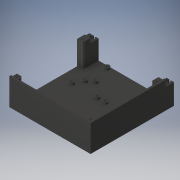
# Autodesk Inventor part: Base Right No Front Panel Or Back Panel
Saved by Autodesk Inventor 2019 (Build 230136000, 136)
## iProperties
Created: 2018-11-05
Part Number: Base Right No Front Panel Or Back Panel
Material: Generic
Document SubType Name: Modeling
Designer: Keith
Density: 1 g/cm^3
Appearance: Default
Author: Keith
## iProperties of the stored document Base Right No Front Panel_3DPrint.ipt
Created: 2018-12-04
Part Number: Base Right No Front Panel_3DPrint
Material: Generic
Document SubType Name: Modeling
Designer: Keith
Density: 1 g/cm^3
Appearance: Default
Author: Keith
Autodesk Inventor part; units mm, degrees
ref_plane "YZ Plane" through (0, 0, 0) normal (1, 0, 0) x (0, 1, 0)
ref_plane "XZ Plane" through (0, 0, 0) normal (0, 1, 0) x (-1, 0, 0)
sketch "Sketch1" plane through (0, 0, 0) normal (0, 1, 0) x (-1, 0, 0)
  line L0 (0, 0) -> (124, 0)
  line L1 (124, 0) -> (124, -124.8)
  line L2 (0, -124.8) -> (0, 0)
  line L3 (113, -2.5) -> (11, -2.5)
  line L4 (124, 0) -> (113, 0)
  line L5 (113, -2.5) -> (113, -11.25)
  line L6 (113, -11.25) -> (121.5, -11.25)
  line L7 (124, -11.25) -> (124, 0)
  line L8 (0, 0) -> (11, 0)
  line L9 (11, -2.5) -> (11, -11.25)
  line L10 (11, -11.25) -> (2.5, -11.25)
  line L11 (0, -11.25) -> (0, 0)
  line L12 (113, -112.8) -> (121.5, -112.8)
  line L13 (124, -112.8) -> (124, -124.8)
  line L14 (11, -112.8) -> (2.5, -112.8)
  line L15 (0, -112.8) -> (0, -124.8)
  line L16 (2.5, -112.8) -> (11, -112.8)
  line L17 (11, -112.8) -> (11, -101.55)
  line L18 (11, -101.55) -> (2.5, -101.55)
  line L19 (0, -101.55) -> (0, -112.8)
  line L20 (113, -112.8) -> (121.5, -112.8)
  line L21 (124, -112.8) -> (124, -101.55)
  line L22 (121.5, -101.55) -> (113, -101.55)
  line L23 (113, -101.55) -> (113, -112.8)
  line L24 (2.5, -11.25) -> (2.5, -101.55)
  line L25 (2.5, -112.8) -> (2.5, -122.3)
  line L26 (121.5, -122.3) -> (121.5, -112.8)
  line L27 (121.5, -101.55) -> (121.5, -11.25)
  line L28 (121.5, -122.3) -> (121.5, -124.8)
  line L29 (2.5, -122.3) -> (2.5, -124.8)
  line L30 (124, -124.8) -> (121.5, -124.8)
  line L31 (2.5, -124.8) -> (0, -124.8)
  dimension "d1" = 124.8
  dimension "d3" = 2.5
  dimension "d6" = 11
  dimension "d7" = 11.25
  dimension "d8" = 11
  dimension "d9" = 11.25
  dimension "d10" = 11
  dimension "d12" = 11
  dimension "d14" = 11
  dimension "d15" = 11.25
  dimension "d16" = 11.25
  constraints: 64 end point, 15 parallel, 9 perpendicular, 6 horizontal, 1 point on line
  measures "d1" distance of L0.end L1.end
  measures "d3" distance between parallel lines of L0 L3
  measures "d6" distance of L7.start L5.end
  measures "d7" distance of L5.end L4.end
  measures "d8" distance of L9.end L11.start
  measures "d9" distance of L8.end L9.end
  measures "d10" distance of L12.start L13.start
  measures "d12" distance of L15.start L14.start
  measures "d14" distance of L19.start L17.end
  measures "d15" distance of L17.end L16.end
  measures "d16" distance of L21.end L21.start
extrude "Extrusion1" add sketch "Sketch1" along normal blind 43
sketch "Sketch2" plane through (0, 0, 0) normal (0, -1, 0) x (1, 0, 0)
  line L0 (0, 0) -> (0, -124.8) projected
  line L1 (-124, 0) -> (0, 0) projected
  line L2 (-124, -124.8) -> (-124, 0) projected
  line L3 (-121.5, -124.8) -> (-124, -124.8) projected
  line L4 (-121.5, -112.8) -> (-121.5, -124.8) projected
  line L5 (-113, -112.8) -> (-121.5, -112.8) projected
  line L6 (-113, -101.55) -> (-113, -112.8) projected
  line L7 (-121.5, -101.55) -> (-113, -101.55) projected
  line L8 (-121.5, -11.25) -> (-121.5, -101.55) projected
  line L9 (-113, -11.25) -> (-121.5, -11.25) projected
  line L10 (-113, -2.5) -> (-113, -11.25) projected
  line L11 (-11, -2.5) -> (-113, -2.5) projected
  line L12 (-11, -11.25) -> (-11, -2.5) projected
  line L13 (-2.5, -11.25) -> (-11, -11.25) projected
  line L14 (-2.5, -101.55) -> (-2.5, -11.25) projected
  line L15 (-11, -101.55) -> (-2.5, -101.55) projected
  line L16 (-11, -112.8) -> (-11, -101.55) projected
  line L17 (-2.5, -112.8) -> (-11, -112.8) projected
  line L18 (-2.5, -124.8) -> (-2.5, -112.8) projected
  line L19 (0, -124.8) -> (-2.5, -124.8) projected
  line L20 (-124, -124.8) -> (0, -124.8)
  line L21 (0, -124.8) -> (0, 0)
  line L22 (0, 0) -> (-124, 0)
  line L23 (-124, 0) -> (-124, -124.8)
  constraints: 8 end point, 2 parallel, 1 horizontal, 1 perpendicular
extrude "Extrusion2" add sketch "Sketch2" against normal blind 2
sketch "Sketch3" plane through (0, 2, 0) normal (0, 1, 0) x (1, 0, 0)
  line L0 (-121.5, 112.8) -> (-121.5, 124.8) projected
  line L1 (-113, 112.8) -> (-121.5, 112.8) projected
  line L2 (-113, 101.55) -> (-113, 112.8) projected
  line L3 (-121.5, 101.55) -> (-113, 101.55) projected
  line L4 (-121.5, 11.25) -> (-121.5, 101.55) projected
  line L5 (-113, 11.25) -> (-121.5, 11.25) projected
  line L6 (-113, 2.5) -> (-113, 11.25) projected
  line L7 (-11, 2.5) -> (-113, 2.5) projected
  line L8 (-11, 11.25) -> (-11, 2.5) projected
  line L9 (-2.5, 11.25) -> (-11, 11.25) projected
  line L10 (-2.5, 101.55) -> (-2.5, 11.25) projected
  line L11 (-11, 101.55) -> (-2.5, 101.55) projected
  line L12 (-11, 112.8) -> (-11, 101.55) projected
  line L13 (-2.5, 112.8) -> (-11, 112.8) projected
  line L14 (-2.5, 124.8) -> (-2.5, 112.8) projected
  line L15 (-2.5, 124.8) -> (-121.5, 124.8) projected
  line L16 (-11, 112.8) -> (-2.5, 112.8)
  line L17 (-2.5, 112.8) -> (-2.5, 124.8)
  line L18 (-2.5, 124.8) -> (-11, 124.8)
  line L19 (-11, 124.8) -> (-11, 112.8)
  line L20 (-113, 112.8) -> (-121.5, 112.8)
  line L21 (-121.5, 112.8) -> (-121.5, 124.8)
  line L22 (-121.5, 124.8) -> (-113, 124.8)
  line L23 (-113, 124.8) -> (-113, 112.8)
  point P0 (0, 0)
  constraints: 16 end point, 4 parallel, 2 horizontal, 2 perpendicular
extrude "Extrusion3" add sketch "Sketch3" along normal blind 30.6 contours L0 L15 L23 L1 | L15 L14 L13 L19
sketch "Sketch4" plane through (0, 0, -124.8) normal (1, 0, 0) x (0, 0, -1)
  line L0 (0, 32.6) -> (-12, 32.6) projected
  line L1 (-12, 32.6) -> (-12, 43) projected
  line L2 (-124.8, 43) -> (0, 43) projected
  line L3 (0, 0) -> (0, 43) projected
  point P0 (-124.8, 0)
extrude "Extrusion4" cut sketch "Sketch4" against normal through all
sketch "Sketch5" plane through (0, 43, 0) normal (0, 1, 0) x (1, 0, 0)
  line L0 (-113, 112.8) -> (-124, 112.8) projected
  line L1 (-124, 112.8) -> (-124, 0) projected
  line L2 (-124, 0) -> (0, 0) projected
  line L3 (0, 0) -> (0, 112.8) projected
  line L4 (0, 112.8) -> (-11, 112.8) projected
  line L5 (-11, 112.8) -> (-11, 101.55) projected
  line L6 (-11, 101.55) -> (-2.5, 101.55) projected
  line L7 (-2.5, 101.55) -> (-2.5, 11.25) projected
  line L8 (-2.5, 11.25) -> (-11, 11.25) projected
  line L9 (-11, 11.25) -> (-11, 2.5) projected
  line L10 (-11, 2.5) -> (-113, 2.5) projected
  line L11 (-113, 2.5) -> (-113, 11.25) projected
  line L12 (-113, 11.25) -> (-121.5, 11.25) projected
  line L13 (-121.5, 11.25) -> (-121.5, 101.55) projected
  line L14 (-121.5, 101.55) -> (-113, 101.55) projected
  line L15 (-113, 101.55) -> (-113, 112.8) projected
  circle A0 centre (-6.625, 6.875) radius 1.35
  circle A1 centre (-6.625, 105.8) radius 1.35
  line L16 (-62, 2.5) -> (-62, 12.6966)
  line L17 (0, 0) -> (-124, 0)
  line L18 (-124, 0) -> (-124, 112.8)
  line L19 (-124, 112.8) -> (-113, 112.8)
  line L20 (-113, 112.8) -> (-113, 101.55)
  line L21 (-113, 101.55) -> (-121.5, 101.55)
  line L22 (-121.5, 101.55) -> (-121.5, 11.25)
  line L23 (-121.5, 11.25) -> (-113, 11.25)
  line L24 (-113, 11.25) -> (-113, 2.5)
  line L25 (-113, 2.5) -> (-11, 2.5)
  circle A2 centre (-117.375, 6.875) radius 1.35
  circle A3 centre (-117.375, 105.8) radius 1.35
  dimension "d25" = 2.7
  dimension "d26" = 4.375
  dimension "d27" = 4.375
  dimension "d28" = 2.7
  dimension "d29" = 4.25
  dimension "d30" = 4.375
  constraints: 20 end point, 7 symmetric about line, 4 centre point, 1 midpoint, 1 vertical, 2 other
  measures "d25" diameter of A0
  measures "d26" distance from line of L8 A0.centre
  measures "d27" distance from line of L9 A0.centre
  measures "d28" diameter of A1
  measures "d29" distance from line of L6 A1.centre
  measures "d30" distance from line of L5 A1.centre
extrude "Extrusion5" cut sketch "Sketch5" against normal blind 12 contours A0 | A1 | A2 | A3
sketch "Sketch6" plane through (0, 0, 0) normal (1, 0, 0) x (0, 0, -1)
  line L0 (0, 43) -> (112.8, 43) projected
  line L1 (0, 0) -> (0, 43) projected
  line L2 (0, 0) -> (124.8, 0) projected
  line L3 (124.8, 0) -> (124.8, 32.6) projected
  line L4 (112.8, 32.6) -> (112.8, 43) projected
  line L5 (124.8, 0) -> (124.8, 32.6) projected
  line L6 (112.8, 32.6) -> (124.8, 32.6)
  line L7 (124.8, 32.6) -> (124.8, 30.6)
  line L8 (124.8, 30.6) -> (112.8, 30.6)
  line L9 (112.8, 30.6) -> (112.8, 32.6)
  line L10 (124.8, 32.6) -> (112.8, 32.6) projected
  line L11 (112.8, 32.6) -> (112.8, 43) projected
  dimension "d33" = 30.6
  constraints: 8 end point, 2 parallel, 1 horizontal, 1 perpendicular, 1 point on line
  measures "d33" distance between parallel lines of L2 L8
extrude "Extrusion6" cut sketch "Sketch6" against normal through all contours L6 L3 L8 L9
sketch "Sketch7" plane through (0, 43, 0) normal (0, 1, 0) x (1, 0, 0)
  circle A0 centre (-6.625, 6.875) radius 1.35 projected
  circle A1 centre (-117.375, 105.8) radius 1.35 projected
  circle A2 centre (-6.625, 6.875) radius 1.35 projected
  circle A3 centre (-6.625, 105.8) radius 1.35 projected
  circle A4 centre (-117.375, 6.875) radius 1.35 projected
  line L0 (-113, 112.8) -> (-124, 112.8) projected
  line L1 (-124, 112.8) -> (-124, 0) projected
  line L2 (-124, 0) -> (0, 0) projected
  line L3 (0, 0) -> (0, 112.8) projected
  line L4 (0, 112.8) -> (-11, 112.8) projected
  line L5 (-11, 112.8) -> (-11, 101.55) projected
  line L6 (-11, 101.55) -> (-2.5, 101.55) projected
  line L7 (-2.5, 101.55) -> (-2.5, 11.25) projected
  line L8 (-2.5, 11.25) -> (-11, 11.25) projected
  line L9 (-11, 11.25) -> (-11, 2.5) projected
  line L10 (-11, 2.5) -> (-113, 2.5) projected
  line L11 (-113, 2.5) -> (-113, 11.25) projected
  line L12 (-113, 11.25) -> (-121.5, 11.25) projected
  line L13 (-121.5, 11.25) -> (-121.5, 101.55) projected
  line L14 (-121.5, 101.55) -> (-113, 101.55) projected
  line L15 (-113, 101.55) -> (-113, 112.8) projected
extrude "Extrusion7" cut sketch "Sketch7" against normal blind 3
sketch "Sketch8" plane through (0, 30.6, -112.8) normal (0, 1, 0) x (1, 0, 0)
  line L0 (-113, 12) -> (-113, 0) projected
  line L1 (-124, 12) -> (-113, 12) projected
  line L2 (-124, 0) -> (-124, 12) projected
  line L3 (-113, 0) -> (-124, 0) projected
  line L4 (-11, 0) -> (-11, 12) projected
  line L5 (0, 0) -> (-11, 0) projected
  line L6 (0, 12) -> (0, 0) projected
  line L7 (-11, 12) -> (0, 12) projected
  line L8 (-122.6, 10.6) -> (-122.6, 9.3834)
  line L9 (-120.075, 10.6) -> (-122.6, 10.6)
  line L10 (-122.6, 9.3834) -> (-120.0827, 6.9051)
  line L11 (-114.4, 10.6) -> (-114.4, 9.3834)
  line L12 (-116.925, 10.6) -> (-114.4, 10.6)
  line L13 (-114.4, 9.3834) -> (-116.9173, 6.9051)
  line L14 (-120, 12) -> (-117, 12)
  line L15 (-120.0827, 6.9051) -> (-116.9173, 6.9051)
  line L16 (-120.075, 10.6) -> (-120.075, 12)
  line L17 (-116.925, 10.6) -> (-116.925, 12)
  line L18 (-120.075, 12) -> (-120, 12)
  line L19 (0, 12) -> (-124, 12) projected
  line L20 (-117, 12) -> (-116.925, 12)
  point P0 (0, -112.8)
  point P1 (-114.4, 9.9917)
  constraints: 24 end point, 5 horizontal, 4 vertical, 3 collinear, 3 point on line, 1 midpoint, 3 other
extrude "Extrusion8" cut sketch "Sketch8" against normal through all contours L17 L12 L11 L13 L15 L10 L8 L9 L16 L1
ref_plane "Work Plane1" through (-62, 2, -101.55) normal (1, 0, 0) x (0, 0, -1)
mirror "Mirror1" about plane through (-62, 2, -101.55) normal (1, 0, 0) of "Extrusion8"
sketch "Sketch9" plane through (-124, 0, -124.8) normal (-1, 0, 0) x (0, 0, 1)
  line L0 (124.8, 40) -> (12, 40) projected
  line L1 (12, 40) -> (12, 30.6) projected
  line L2 (12, 30.6) -> (0, 30.6) projected
  line L3 (0, 0) -> (0, 30.6) projected
  line L4 (0, 0) -> (124.8, 0) projected
  line L5 (124.8, 0) -> (124.8, 40) projected
  line L6 (124.8, 40) -> (164.8, 40)
  line L7 (164.8, 40) -> (164.8, 0)
  line L8 (164.8, 0) -> (124.8, 0)
  line L9 (124.8, 0) -> (124.8, 40)
  circle A0 centre (134.8, 30) radius 2.6
  circle A1 centre (154.8, 30) radius 2.6
  circle A2 centre (154.8, 10) radius 2.6
  circle A3 centre (134.8, 10) radius 2.6
  dimension "d61" = 40
  dimension "d62" = 5.2
  dimension "d63" = 5.2
  dimension "d64" = 5.2
  dimension "d65" = 5.2
  dimension "d66" = 20
  dimension "d67" = 20
  dimension "d68" = 20
  dimension "d69" = 10
  dimension "d141" = 10
  dimension "d142" = 10
  dimension "d143" = 10
  constraints: 8 end point, 4 centre point, 2 parallel, 1 horizontal, 1 perpendicular
  measures "d61" distance of L7.end L8.end
  measures "d62" diameter of A0
  measures "d63" diameter of A1
  measures "d64" diameter of A2
  measures "d65" diameter of A3
  measures "d66" distance of A1.centre A0.centre
  measures "d67" distance of A2.centre A3.centre
  measures "d68" distance between centres of A1 A2
  measures "d69" distance from line of L8 A3.centre
  measures "d141" distance from line of L5 A0.centre
  measures "d142" distance from line of L6 A0.centre
  measures "d143" distance from line of L5 A3.centre
extrude "Extrusion9" add sketch "Sketch9" along normal blind 2.5
sketch "Sketch10" plane through (0, 2, 0) normal (0, 1, 0) x (1, 0, 0)
  line L0 (-113, 124.8) -> (-113, 101.55) projected
  line L1 (-121.5, 101.55) -> (-113, 101.55) projected
  line L2 (-121.5, 11.25) -> (-121.5, 101.55) projected
  line L3 (-113, 11.25) -> (-121.5, 11.25) projected
  line L4 (-113, 2.5) -> (-113, 11.25) projected
  line L5 (-11, 2.5) -> (-113, 2.5) projected
  line L6 (-11, 11.25) -> (-11, 2.5) projected
  line L7 (-2.5, 11.25) -> (-11, 11.25) projected
  line L8 (-2.5, 101.55) -> (-2.5, 11.25) projected
  line L9 (-11, 101.55) -> (-2.5, 101.55) projected
  line L10 (-11, 124.8) -> (-11, 101.55) projected
  line L11 (-11, 124.8) -> (-113, 124.8) projected
  circle A0 centre (-20.1, 87.8) radius 3.5
  circle A1 centre (-96.1, 87.8) radius 3.5
  line L12 (0, 112.8) -> (0, 0) projected
  circle A2 centre (-20.1, 87.8) radius 1.35
  circle A3 centre (-96.1, 87.8) radius 1.35
  dimension "d72" = 7
  dimension "d73" = 7
  dimension "d74" = 76
  dimension "d76" = 37
  dimension "d77" = 20.1
  dimension "d78" = 2.7
  dimension "d79" = 2.7
  constraints: 4 centre point, 2 coincident
  measures "d72" diameter of A0
  measures "d73" diameter of A1
  measures "d74" distance of A0.centre A1.centre
  measures "d76" distance from line of L11 A0.centre
  measures "d77" distance from line of L12 A0.centre
  measures "d78" diameter of A2
  measures "d79" diameter of A3
extrude "Extrusion10" add sketch "Sketch10" along normal blind 3 contours A0 | A1
sketch "Sketch11" plane through (0, 2, 0) normal (0, 1, 0) x (1, 0, 0)
  circle A0 centre (-20.1, 87.8) radius 1.35 projected
  circle A1 centre (-96.1, 87.8) radius 1.35 projected
  point P0 (0, 0)
extrude "Extrusion11" cut sketch "Sketch11" against normal blind 1
sketch "Sketch12" plane through (0, 2, 0) normal (0, 1, 0) x (1, 0, 0)
  circle A0 centre (-20.1, 87.8) radius 3.5 projected
  circle A1 centre (-96.1, 87.8) radius 3.5 projected
  line L0 (-113, 124.8) -> (-113, 101.55) projected
  line L1 (-121.5, 101.55) -> (-113, 101.55) projected
  line L2 (-121.5, 11.25) -> (-121.5, 101.55) projected
  line L3 (-113, 11.25) -> (-121.5, 11.25) projected
  line L4 (-113, 2.5) -> (-113, 11.25) projected
  line L5 (-11, 2.5) -> (-113, 2.5) projected
  line L6 (-11, 11.25) -> (-11, 2.5) projected
  line L7 (-2.5, 11.25) -> (-11, 11.25) projected
  line L8 (-2.5, 101.55) -> (-2.5, 11.25) projected
  line L9 (-11, 101.55) -> (-2.5, 101.55) projected
  line L10 (-11, 124.8) -> (-11, 101.55) projected
  line L11 (-11, 124.8) -> (-113, 124.8) projected
  circle A2 centre (-103, 12.5) radius 3.5
  circle A3 centre (-103, 75.3) radius 3.5
  circle A4 centre (-65.2, 12.5) radius 3.5
  circle A5 centre (-65.2, 75.3) radius 3.5
  circle A6 centre (-103, 12.5) radius 1.35
  circle A7 centre (-103, 75.3) radius 1.35
  circle A8 centre (-65.2, 75.3) radius 1.35
  circle A9 centre (-65.2, 12.5) radius 1.35
  line L12 (-59.1, 6.875) -> (-59.1, 19.1596)
  circle A10 centre (-15.2, 12.5) radius 3.5
  circle A11 centre (-15.2, 75.3) radius 3.5
  circle A12 centre (-53, 12.5) radius 3.5
  circle A13 centre (-53, 75.3) radius 3.5
  circle A14 centre (-15.2, 12.5) radius 1.35
  circle A15 centre (-15.2, 75.3) radius 1.35
  circle A16 centre (-53, 75.3) radius 1.35
  circle A17 centre (-53, 12.5) radius 1.35
  point P0 (0, 0)
  dimension "d84" = 7
  dimension "d85" = 7
  dimension "d86" = 7
  dimension "d87" = 7
  dimension "d88" = 62.8
  dimension "d89" = 62.8
  dimension "d90" = 37.8
  dimension "d91" = 10
  dimension "d92" = 10
  dimension "d93" = 2.7
  dimension "d94" = 2.7
  dimension "d95" = 2.7
  dimension "d96" = 2.7
  dimension "d97" = 6.1
  constraints: 16 centre point, 8 coincident, 8 symmetric about line, 2 end point, 1 vertical, 8 other
  measures "d84" diameter of A2
  measures "d85" diameter of A3
  measures "d86" diameter of A4
  measures "d87" diameter of A5
  measures "d88" distance of A3.centre A2.centre
  measures "d89" distance of A5.centre A4.centre
  measures "d90" distance of A4.centre A2.centre
  measures "d91" distance from line of L5 A2.centre
  measures "d92" distance from line of L4 A2.centre
  measures "d93" diameter of A6
  measures "d94" diameter of A7
  measures "d95" diameter of A8
  measures "d96" diameter of A9
  measures "d97" distance from line of A9.centre L12
extrude "Extrusion12" add sketch "Sketch12" along normal blind 3 contours A2 | A3 | A4 | A5 | A10 | A11 | A12 | A13
sketch "Sketch13" plane through (0, 2, 0) normal (0, 1, 0) x (1, 0, 0)
  circle A0 centre (-103, 12.5) radius 1.35 projected
  circle A1 centre (-103, 75.3) radius 1.35 projected
  circle A2 centre (-65.2, 75.3) radius 1.35 projected
  circle A3 centre (-65.2, 12.5) radius 1.35 projected
  circle A4 centre (-53, 12.5) radius 1.35 projected
  circle A5 centre (-53, 75.3) radius 1.35 projected
  circle A6 centre (-15.2, 75.3) radius 1.35 projected
  circle A7 centre (-15.2, 12.5) radius 1.35 projected
  point P0 (0, 0)
extrude "Extrusion13" cut sketch "Sketch13" against normal blind 1
sketch "Sketch15" plane through (0, 40, 0) normal (0, 1, 0) x (1, 0, 0)
  circle A0 centre (-117.375, 6.875) radius 1.35 projected
  circle A1 centre (-6.625, 105.8) radius 1.35 projected
  circle A2 centre (-117.375, 105.8) radius 1.35 projected
  circle A3 centre (-6.625, 6.875) radius 1.35 projected
  line L0 (-126.5, 112.8) -> (-113, 112.8) projected
  line L1 (-126.5, -40) -> (-126.5, 112.8) projected
  line L2 (-124, -40) -> (-126.5, -40) projected
  line L3 (-124, -40) -> (-124, 0) projected
  line L4 (0, 0) -> (-124, 0) projected
  line L5 (0, 112.8) -> (0, 0) projected
  line L6 (-11, 112.8) -> (0, 112.8) projected
  line L7 (-11, 101.55) -> (-11, 112.8) projected
  line L8 (-2.5, 101.55) -> (-11, 101.55) projected
  line L9 (-2.5, 11.25) -> (-2.5, 101.55) projected
  line L10 (-11, 11.25) -> (-2.5, 11.25) projected
  line L11 (-11, 2.5) -> (-11, 11.25) projected
  line L12 (-113, 2.5) -> (-11, 2.5) projected
  line L13 (-113, 11.25) -> (-113, 2.5) projected
  line L14 (-121.5, 11.25) -> (-113, 11.25) projected
  line L15 (-121.5, 101.55) -> (-121.5, 11.25) projected
  line L16 (-113, 101.55) -> (-121.5, 101.55) projected
  line L17 (-113, 112.8) -> (-113, 101.55) projected
  line L18 (-121.5, 2.5) -> (-2.5, 2.5)
  line L19 (-2.5, 2.5) -> (-2.5, 112.8)
  line L20 (-2.5, 112.8) -> (-121.5, 112.8)
  line L21 (-121.5, 112.8) -> (-121.5, 2.5)
  constraints: 8 end point, 2 parallel, 1 horizontal, 1 perpendicular, 1 point on line
extrude "Extrusion15" cut sketch "Sketch15" against normal blind 2.5 contours L0 L17 L16 L21 | L20 L7 L8 L9 L10 L11 L12 L13 L14 L15 L16 L17 | L6 L19 L8 L7 | L14 L13 L18 L21 | L19 L18 L11 L10
fillet "Fillet2" radius 3 4 edges at (-11, 19.75, -101.55) (-11, 19.75, -11.25) (-113, 19.75, -101.55) (-113, 19.75, -11.25)
sketch "Sketch16" plane through (0, 2, 0) normal (0, 1, 0) x (1, 0, 0)
  line L0 (-11, 124.8) -> (-113, 124.8) projected
  arc A0 (-8, 11.25) -> (-11, 8.25) centre (-8, 8.25) ccw projected
  line L1 (-2.5, 11.25) -> (-8, 11.25) projected
  line L2 (-2.5, 101.55) -> (-2.5, 11.25) projected
  line L3 (-8, 101.55) -> (-2.5, 101.55) projected
  arc A1 (-11, 104.55) -> (-8, 101.55) centre (-8, 104.55) ccw projected
  line L4 (-11, 124.8) -> (-11, 104.55) projected
  line L5 (-11, 124.8) -> (-113, 124.8) projected
  line L6 (-113, 124.8) -> (-113, 104.55) projected
  arc A2 (-116, 101.55) -> (-113, 104.55) centre (-116, 104.55) ccw projected
  line L7 (-121.5, 101.55) -> (-116, 101.55) projected
  line L8 (-121.5, 11.25) -> (-121.5, 101.55) projected
  line L9 (-116, 11.25) -> (-121.5, 11.25) projected
  arc A3 (-113, 8.25) -> (-116, 11.25) centre (-116, 8.25) ccw projected
  line L10 (-113, 2.5) -> (-113, 8.25) projected
  line L11 (-11, 2.5) -> (-113, 2.5) projected
  line L12 (-11, 8.25) -> (-11, 2.5) projected
  circle A4 centre (-20.1, 120.8) radius 3.5
  circle A5 centre (-96.1, 120.8) radius 3.5
  circle A6 centre (-20.1, 120.8) radius 1.35
  circle A7 centre (-96.1, 120.8) radius 1.35
  point P0 (0, 0)
  dimension "d132" = 7
  dimension "d133" = 7
  dimension "d134" = 76
  dimension "d136" = 2.7
  dimension "d137" = 2.7
  constraints: 4 centre point, 2 coincident
  measures "d132" diameter of A4
  measures "d133" diameter of A5
  measures "d134" distance of A5.centre A4.centre
  measures "d136" diameter of A6
  measures "d137" diameter of A7
extrude "Extrusion16" add sketch "Sketch16" along normal blind 3 contours A4 | A5
sketch "Sketch19" plane through (-126.5, 0, -124.8) normal (-1, 0, 0) x (0, 0, 1)
  circle A0 centre (134.8, 10) radius 2.6 projected
  circle A1 centre (154.8, 10) radius 2.6 projected
  circle A2 centre (154.8, 30) radius 2.6 projected
  circle A3 centre (134.8, 30) radius 2.6 projected
  line L0 (0, 0) -> (164.8, 0) projected
  line L1 (164.8, 0) -> (164.8, 40) projected
  line L2 (164.8, 40) -> (12, 40) projected
  line L3 (12, 40) -> (12, 30.6) projected
  line L4 (12, 30.6) -> (0, 30.6) projected
  line L5 (0, 30.6) -> (0, 0) projected
  line L6 (164.8, 40) -> (12, 40) projected
  line L7 (12, 40) -> (164.8, 40)
  line L8 (164.8, 40) -> (164.8, 0)
  line L9 (164.8, 0) -> (12, 0)
  line L10 (12, 0) -> (12, 40)
  point P0 (124.8, 0)
  dimension "d156" = 152.8
  dimension "d157" = 40
  constraints: 8 end point, 2 parallel, 1 horizontal, 1 perpendicular
  measures "d156" distance of L1.end L2.end
  measures "d157" distance of L7.end L0.end
extrude "Extrusion18" cut sketch "Sketch19" against normal blind 5 contours A0 | A1 | A2 | A3 | L10 L3 L2 L1 L0
sketch "Sketch20" plane through (-121.5, 0, -124.8) normal (-1, 0, 0) x (0, 0, 1)
  line L0 (23.25, 37.5) -> (12, 37.5) projected
  line L1 (12, 30.6) -> (12, 37.5) projected
  line L2 (12, 0) -> (12, 30.6) projected
  line L3 (124.8, 0) -> (12, 0) projected
  line L4 (124.8, 40) -> (124.8, 0) projected
  line L5 (122.3, 40) -> (124.8, 40) projected
  line L6 (122.3, 40) -> (122.3, 37.5) projected
  line L7 (122.3, 37.5) -> (113.55, 37.5) projected
  line L8 (113.55, 2) -> (113.55, 37.5) projected
  line L9 (113.55, 2) -> (23.25, 2) projected
  line L10 (23.25, 2) -> (23.25, 37.5) projected
  circle A0 centre (17.625, 27.5) radius 1.35
  circle A1 centre (17.625, 10) radius 1.35
  circle A2 centre (117.925, 27.5) radius 1.35
  circle A3 centre (118.3451, 10) radius 1.35
  dimension "d160" = 2.7
  dimension "d161" = 2.7
  dimension "d162" = 10
  dimension "d163" = 10
  dimension "d164" = 2.7
  dimension "d165" = 2.7
  dimension "d168" = 5.625
  constraints: 4 centre point
  measures "d160" diameter of A0
  measures "d161" diameter of A1
  measures "d162" distance from line of L3 A1.centre
  measures "d163" distance from line of L0 A0.centre
  measures "d164" diameter of A2
  measures "d165" diameter of A3
  measures "d168" distance from line of L1 A0.centre
extrude "Extrusion19" cut sketch "Sketch20" against normal blind 6 contours A0 | A1 | A2 | A3
sketch "Sketch21" plane through (0, 2, 0) normal (0, 1, 0) x (1, 0, 0)
  line L0 (-11, 124.8) -> (-113, 124.8) projected
  line L1 (-113, 124.8) -> (-113, 104.55) projected
  arc A0 (-116, 101.55) -> (-113, 104.55) centre (-116, 104.55) ccw projected
  line L2 (-121.5, 101.55) -> (-116, 101.55) projected
  line L3 (-121.5, 11.25) -> (-121.5, 101.55) projected
  line L4 (-116, 11.25) -> (-121.5, 11.25) projected
  arc A1 (-113, 8.25) -> (-116, 11.25) centre (-116, 8.25) ccw projected
  line L5 (-113, 2.5) -> (-113, 8.25) projected
  line L6 (-11, 2.5) -> (-113, 2.5) projected
  line L7 (-11, 8.25) -> (-11, 2.5) projected
  arc A2 (-8, 11.25) -> (-11, 8.25) centre (-8, 8.25) ccw projected
  line L8 (-2.5, 11.25) -> (-8, 11.25) projected
  line L9 (-2.5, 101.55) -> (-2.5, 11.25) projected
  line L10 (-8, 101.55) -> (-2.5, 101.55) projected
  arc A3 (-11, 104.55) -> (-8, 101.55) centre (-8, 104.55) ccw projected
  line L11 (-11, 124.8) -> (-11, 104.55) projected
  circle A4 centre (-20.1, 94.6) radius 3.5
  circle A5 centre (-87.1, 94.6) radius 3.5
  circle A6 centre (-20.1, 120.8) radius 3.5 projected
  circle A7 centre (-20.1, 94.6) radius 1.35
  circle A8 centre (-87.1, 94.6) radius 1.35
  point P0 (0, 0)
  dimension "d170" = 7
  dimension "d172" = 67
  dimension "d175" = 0
  dimension "d176" = 2.7
  dimension "d177" = 2.7
  dimension "d180" = 7
  constraints: 4 centre point, 2 coincident
  measures "d170" diameter of A5
  measures "d172" distance of A5.centre A4.centre
  measures "d175" horizontal distance of A6.centre A4.centre
  measures "d176" diameter of A7
  measures "d177" diameter of A8
  measures "d180" diameter of A4
extrude "Extrusion20" add sketch "Sketch21" along normal blind 3 contours A4 | A5
sketch "Sketch22" plane through (0, 5, 0) normal (0, 1, 0) x (1, 0, 0)
  circle A0 centre (-87.1, 94.6) radius 1.35 projected
  circle A1 centre (-87.1, 94.6) radius 3.5 projected
  circle A2 centre (-20.1, 94.6) radius 1.35 projected
  arc A3 (-20.9307, 91.2) -> (-19.2693, 91.2) centre (-20.1, 87.8) ccw projected
  arc A4 (-19.2693, 91.2) -> (-20.9307, 91.2) centre (-20.1, 94.6) ccw projected
  circle A5 centre (-20.1, 87.8) radius 1.35 projected
  point P0 (0, 0)
extrude "Extrusion21" cut sketch "Sketch22" against normal blind 4 contours A0 | A2
body "Solid1"
